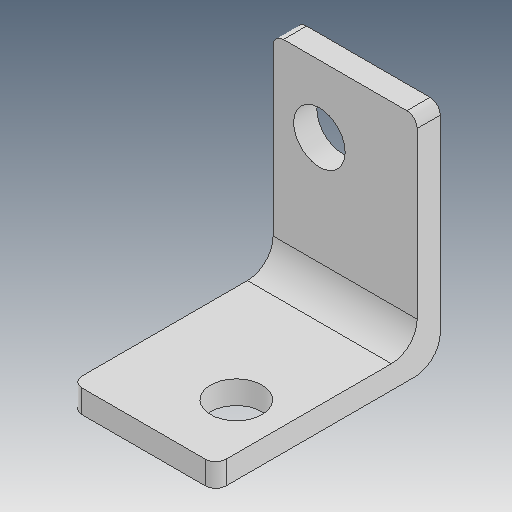
# Autodesk Inventor part: shin_L_bracket
Saved by Autodesk Inventor 2025.2 (Build 292293000, 293)
## iProperties
Created: 2025-02-16
Part Number: shin_L_bracket
Material: Generic
Document SubType Name: Modeling
Designer: email
Density: 1 g/cm^3
Appearance: Default
Author: email
Autodesk Inventor part; units mm, degrees
ref_plane "YZ Plane" through (0, 0, 0) normal (1, 0, 0) x (0, 1, 0)
ref_plane "XZ Plane" through (0, 0, 0) normal (0, 1, 0) x (-1, 0, 0)
ref_plane "XY Plane" through (0, 0, 0) normal (0, 0, 1) x (1, 0, 0)
sketch "Sketch1" plane through (0, 0, 0) normal (1, 0, 0) x (0, 1, 0)
  line L0 (0, 0) -> (4.5, 0)
  line L1 (4.5, 0) -> (4.5, -39.16)
  line L2 (1.7807, -43.66) -> (0, -43.66)
  line L3 (0, -43.66) -> (0, 0)
  line L4 (0, -43.66) -> (43.6, -43.66)
  line L5 (43.6, -43.66) -> (43.6, -39.16)
  line L6 (43.6, -39.16) -> (4.5, -39.16)
  line L7 (0, -7.4197) -> (0, -43.66)
  dimension "d0" = 43.6
  dimension "d1" = 43.66
  dimension "d2" = 4.5
  dimension "d3" = 4.5
  constraints: 16 end point, 4 parallel, 2 horizontal, 2 perpendicular
  measures "d0" distance of L2.end L4.end
  measures "d1" distance of L2.end L0.start
  measures "d2" distance between parallel lines of L4 L6
  measures "d3" distance between parallel lines of L3 L1
extrude "Extrusion1" add sketch "Sketch1" along normal blind 28
sketch "Sketch2" plane through (0, 4.5, 0) normal (0, 1, 0) x (1, 0, 0)
  circle A0 centre (19, 13) radius 5
  line L0 (28, 39.16) -> (28, 0) projected
  line L1 (0, 0) -> (28, 0) projected
  dimension "d6" = 10
  dimension "d7" = 9
  dimension "d8" = 13
  constraints: 1 centre point
  measures "d6" diameter of A0
  measures "d7" distance from line of L0 A0.centre
  measures "d8" distance from line of L1 A0.centre
sketch "Sketch3" plane through (0, 0, -43.66) normal (0, 0, -1) x (-1, 0, 0)
  circle A0 centre (-9, 30.6) radius 5
  line L0 (0, 0) -> (0, 43.6) projected
  line L1 (0, 43.6) -> (-28, 43.6) projected
  dimension "d9" = 9
  dimension "d10" = 13
  dimension "d11" = 10
  constraints: 1 centre point
  measures "d9" distance from line of L0 A0.centre
  measures "d10" distance from line of L1 A0.centre
  measures "d11" diameter of A0
extrude "Extrusion2" cut sketch "Sketch3" against normal up to next
extrude "Extrusion3" cut sketch "Sketch2" against normal up to next
fillet "Fillet1" radius 2 4 edges at (0, 43.6, -41.41) (28, 43.6, -41.41) (0, 2.25, 0) (28, 2.25, 0)
fillet "Fillet2" radius 5 2 edges at (14, 0, -43.66) (14, 4.5, -39.16)
body "Solid1"
